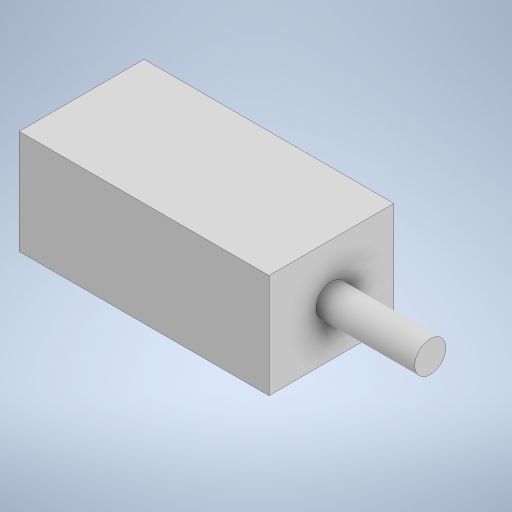
# Autodesk Inventor part: motor
Saved by Autodesk Inventor 2024 (Build 280153020, 153B)
## iProperties
Created: 2023-05-22
Part Number: motor
Material: Generic
Document SubType Name: Modeling
Designer: Diego
Density: 1 g/cm^3
Appearance: Default
Author: Diego
Autodesk Inventor part; units mm, degrees
ref_plane "YZ Plane" through (0, 0, 0) normal (1, 0, 0) x (0, 1, 0)
ref_plane "XZ Plane" through (0, 0, 0) normal (0, 1, 0) x (-1, 0, 0)
ref_plane "XY Plane" through (0, 0, 0) normal (0, 0, 1) x (1, 0, 0)
sketch "Sketch1" plane through (0, 0, 0) normal (0, 1, 0) x (-1, 0, 0)
  line L0 (0, 0) -> (24, 0)
  line L1 (24, 0) -> (24, 12)
  line L2 (24, 12) -> (0, 12)
  line L3 (0, 12) -> (0, 0)
  dimension "d0" = 24
  dimension "d1" = 12
  constraints: 8 end point, 2 parallel, 1 horizontal, 1 perpendicular
  measures "d0" distance of L2.end L1.end
  measures "d1" distance of L1.end L0.end
extrude "Extrusion1" add sketch "Sketch1" along normal blind 10
sketch "Sketch2" plane through (0, 0, 12) normal (1, 0, 0) x (0, 0, -1)
  line L0 (12, 10) -> (0, 10) construction
  line L1 (12, 0) -> (12, 10) construction
  line L2 (0, 10) -> (12, 0) construction
  line L3 (12, 0) -> (0, 0) construction
  line L4 (12, 10) -> (0, 0) construction
  circle A0 centre (6, 5) radius 1.5
  dimension "d4" = 3
  constraints: 4 end point, 1 centre point, 1 midpoint
  measures "d4" diameter of A0
extrude "Extrusion2" add sketch "Sketch2" along normal blind 9.5
body "Solid1"
